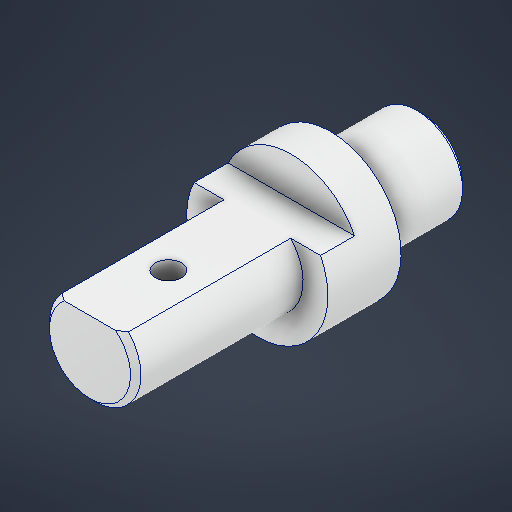
# Autodesk Inventor part: MMAE 232 Assignment 1c-Nicholas Skiba
Saved by Autodesk Inventor 2026.1 (Build 301233000, 233)
## iProperties
Created: 2025-08-25
Part Number: MMAE 232 Assignment 1c-Nicholas Skiba
Material: Aluminum 6061
Document SubType Name: Modeling
Designer: Nick
Density: 2.7 g/cm^3
Appearance: Aluminum - Flat
Mass: 387.404 g
Surface Area: 205.557 cm^2
Volume: 143.483 cm^3
Author: Nick
Autodesk Inventor part; units mm, degrees
ref_plane "XZ Plane" through (0, 0, 0) normal (0, 1, 0) x (-1, 0, 0)
ref_plane "XY Plane" through (0, 0, 0) normal (0, 0, 1) x (1, 0, 0)
sketch "Sketch1" plane through (0, 0, 0) normal (0, 1, 0) x (-1, 0, 0)
  circle A0 centre (0, 0) radius 17.5
  dimension "d0" = 35
  constraints: 1 centre point, 1 coincident
  measures "d0" diameter of A0
extrude "Extrusion1" add sketch "Sketch1" along normal blind 64
sketch "Sketch2" plane through (0, 64, 0) normal (0, 1, 0) x (1, 0, 0)
  circle A0 centre (0, 0) radius 27
  dimension "d3" = 54
  constraints: 1 centre point, 1 coincident
  measures "d3" diameter of A0
extrude "Extrusion2" add sketch "Sketch2" along normal blind 28
sketch "Sketch3" plane through (0, 92, 0) normal (0, 1, 0) x (1, 0, 0)
  circle A0 centre (0, 0) radius 16.65
  dimension "d6" = 33.3
  constraints: 1 centre point, 1 coincident
  measures "d6" diameter of A0
extrude "Extrusion3" add sketch "Sketch3" along normal blind 3
sketch "Sketch4" plane through (0, 95, 0) normal (0, 1, 0) x (1, 0, 0)
  circle A0 centre (0, 0) radius 16.65 projected
  circle A1 centre (0, 0) radius 17.5
  dimension "d9" = 35
  constraints: 1 centre point, 1 coincident
  measures "d9" diameter of A1
extrude "Extrusion4" add sketch "Sketch4" along normal blind 32 contours A0 | A1
ref_plane "Work Plane1" through (27, 64, 0) normal (1, 0, 0) x (0, 1, 0)
sketch "Sketch5" plane through (27, 64, 0) normal (1, 0, 0) x (0, 1, 0)
  line L0 (-64, -17.5) -> (-64, 17.5) projected
  line L1 (-64, -17.5) -> (-64, -50.6158)
  line L2 (-64, -50.6158) -> (13, -50.6158)
  line L3 (13, -50.6158) -> (-82.5223, -50.6158)
  line L4 (-82.5223, -50.6158) -> (-82.5223, 53.8814)
  line L5 (-82.5223, 53.8814) -> (13, 53.8814)
  line L6 (13, 53.8814) -> (13, -50.6158)
  point P0 (-64, 0)
  dimension "d12" = 77
  constraints: 12 end point, 2 parallel, 2 perpendicular, 1 horizontal, 1 vertical
  measures "d12" distance of L1.end L2.end
extrude "Extrusion5" cut sketch "Sketch5" against normal blind 15
sketch "Sketch6" plane through (12, 64, 0) normal (1, 0, 0) x (0, 0, -1)
  line L0 (17.5, -64) -> (-17.5, -64) projected
  line L1 (-17.5, -64) -> (0, -64)
  line L2 (0, -64) -> (0, -34)
  line L3 (0, -34) -> (-17.5, -34)
  line L4 (-17.5, -34) -> (-17.5, -64)
  circle A0 centre (0, -34) radius 5
  point P0 (12.7377, -64)
  point P1 (-12.7377, -64)
  dimension "d15" = 30
  dimension "d16" = 10
  constraints: 8 end point, 2 parallel, 1 centre point, 1 coincident, 1 horizontal, 1 perpendicular
  measures "d15" distance of L2.end L1.end
  measures "d16" diameter of A0
extrude "Extrusion6" cut sketch "Sketch6" against normal through all contours A0 L3 L2 | L2 L3 A0
chamfer "Chamfer1" distance 2 angle 45 2 edges at (-17.5, 0, 0) (-17.5, 127, 0)
body "Solid1"
